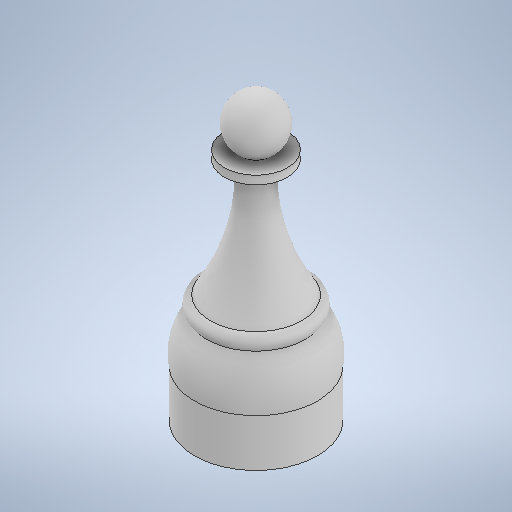
# Autodesk Inventor part: PAWN
Saved by Autodesk Inventor 2025.1 (Build 291241000, 241)
## iProperties
Created: 2024-10-17
Part Number: PAWN
Material: Genérico
Document SubType Name: Modeling
Designer: Octavio
Density: 1 g/cm^3
Appearance: Valor por defecto
Author: Octavio
Autodesk Inventor part; units mm, degrees
ref_plane "YZ Plane" through (0, 0, 0) normal (1, 0, 0) x (0, 1, 0)
ref_plane "XZ Plane" through (0, 0, 0) normal (0, 1, 0) x (-1, 0, 0)
ref_plane "XY Plane" through (0, 0, 0) normal (0, 0, 1) x (1, 0, 0)
sketch "Boceto1" plane through (0, 0, 0) normal (0, 0, 1) x (1, 0, 0)
  line L0 (0, 0) -> (0, 50)
  line L1 (12.9556, 0) -> (0, 0)
  arc A0 (2.2833, 41.1879) -> (0, 50) centre (-0.2888, 45.2233) ccw
  line L2 (2.2833, 41.1879) -> (5.5239, 41.1879)
  line L3 (5.5239, 41.1879) -> (5.5239, 39.7245)
  line L4 (5.5239, 39.7245) -> (2.6625, 39.7245)
  arc A1 (2.6625, 39.7245) -> (7.9966, 19.1386) centre (38.2928, 37.9727) ccw
  arc A2 (8.6471, 16.6281) -> (7.9966, 19.1386) centre (7.7402, 17.7327) ccw
  arc A3 (10.796, 8.3345) -> (8.6471, 16.6281) centre (1.334, 10.308) ccw
  line L5 (10.796, 8.3345) -> (10.796, 0)
  dimension "d0" = 50
  constraints: 12 end point, 8 point on circle, 4 centre point, 4 perpendicular, 1 horizontal, 1 point on line, 1 vertical
  measures "d0" distance of L0.start L0.end
revolve "Revolución1" add sketch "Boceto1" angle 360 about axis through (0, 0, 0) along (0, 1, 0)
